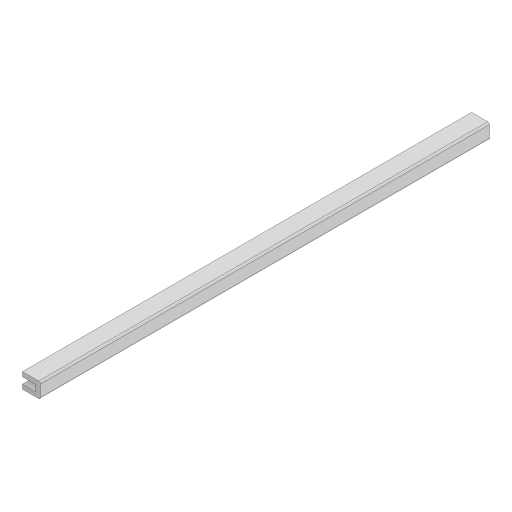
# Autodesk Inventor part: GUIA DE TAPA PRINCIPAL
Saved by Autodesk Inventor 2024 (Build 280153000, 153)
## iProperties
Created: 2024-06-13
Part Number: GUIA DE TAPA PRINCIPAL
Material: Generic
Document SubType Name: Modeling
Designer: Jhuliams
Density: 1 g/cm^3
Appearance: Default
Author: Jhuliams
Autodesk Inventor part; units mm, degrees
ref_plane "YZ Plane" through (0, 0, 0) normal (1, 0, 0) x (0, 1, 0)
ref_plane "XZ Plane" through (0, 0, 0) normal (0, 1, 0) x (-1, 0, 0)
ref_plane "XY Plane" through (0, 0, 0) normal (0, 0, 1) x (1, 0, 0)
sketch "Sketch1" plane through (0, 0, 0) normal (0, 0, 1) x (1, 0, 0)
  line L0 (-7.5, 3.5) -> (7.5, 3.5)
  line L1 (7.5, 3.5) -> (7.5, -3.5)
  line L2 (7.5, -3.5) -> (-7.5, -3.5)
  line L3 (-7.5, -3.5) -> (-7.5, 3.5)
  line L4 (-7.5, 3.5) -> (7.5, -3.5) construction
  line L5 (7.5, 3.5) -> (-7.5, -3.5) construction
  line L6 (-12.5, 8.5) -> (12.5, 8.5)
  line L7 (12.5, 8.5) -> (12.5, -8.5)
  line L8 (12.5, -8.5) -> (-12.5, -8.5)
  line L9 (-12.5, -8.5) -> (-12.5, 8.5)
  line L10 (-12.5, 8.5) -> (12.5, -8.5) construction
  line L11 (12.5, 8.5) -> (-12.5, -8.5) construction
  line L12 (-7.5, 8.5) -> (-7.5, -8.5)
  point P0 (0, 0)
  dimension "d0" = 15
  dimension "d1" = 7
  dimension "d2" = 25
  dimension "d3" = 17
  constraints: 26 end point, 4 midpoint, 4 parallel, 3 perpendicular, 2 horizontal, 2 point on line
  measures "d0" distance of L1.end L2.end
  measures "d1" distance of L0.end L1.end
  measures "d2" distance of L7.end L8.end
  measures "d3" distance of L6.end L7.end
extrude "Extrusion1" add sketch "Sketch1" along normal blind 500 contours L12 L6 L7 L8 L2 L1 L0
fillet "Fillet1" radius 2 2 edges at (12.5, 8.5, 250) (12.5, -8.5, 250)
body "Solid1"
